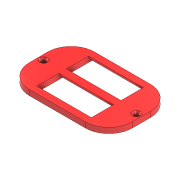
# Autodesk Inventor part: Wago2Din_2Way
Saved by Autodesk Inventor 2021 (Build 250183000, 183)
## iProperties
Created: 2021-07-31
Part Number: Wago2Din_2Way
Material: Generisch
Document SubType Name: Modeling
Designer: Rama
Density: 1 g/cm^3
Appearance: Hellrot
Author: Rama
Autodesk Inventor part; units mm, degrees
ref_plane "YZ Plane" through (0, 0, 0) normal (1, 0, 0) x (0, 1, 0)
ref_plane "XZ Plane" through (0, 0, 0) normal (0, 1, 0) x (-1, 0, 0)
ref_plane "XY Plane" through (0, 0, 0) normal (0, 0, 1) x (1, 0, 0)
sketch "Skizze1" plane through (0, 0, 0) normal (0, 1, 0) x (-1, 0, 0)
  line L0 (15.1, 14.35) -> (-15.1, 14.35)
  line L1 (-15.1, 14.35) -> (-15.1, 2.05)
  line L2 (-15.1, 2.05) -> (15.1, 2.05)
  line L3 (15.1, 2.05) -> (15.1, 14.35)
  line L4 (15.1, 14.35) -> (-15.1, 2.05) construction
  line L5 (-15.1, 14.35) -> (15.1, 2.05) construction
  line L6 (15.1, -2.05) -> (-15.1, -2.05)
  line L7 (-15.1, -2.05) -> (-15.1, -14.35)
  line L8 (-15.1, -14.35) -> (15.1, -14.35)
  line L9 (15.1, -14.35) -> (15.1, -2.05)
  line L10 (15.1, -2.05) -> (-15.1, -14.35) construction
  line L11 (-15.1, -2.05) -> (15.1, -14.35) construction
  line L12 (28.45, 18) -> (-28.45, 18)
  line L13 (-28.45, 18) -> (-28.45, -18)
  line L14 (-28.45, -18) -> (28.45, -18)
  line L15 (28.45, -18) -> (28.45, 18)
  line L16 (28.45, 18) -> (-28.45, -18) construction
  line L17 (-28.45, 18) -> (28.45, -18) construction
  point P0 (0, 0)
  point P1 (0, 8.2)
  point P2 (0, -8.2)
  dimension "d0" = 30.2
  dimension "d1" = 12.3
  dimension "d2" = 30.2
  dimension "d3" = 12.3
  dimension "d5" = 4.1
  dimension "d6" = 2.05
  dimension "d7" = 56.9
  dimension "d8" = 36
  constraints: 36 end point, 6 midpoint, 6 parallel, 3 horizontal, 3 perpendicular
  measures "d0" distance of L2.end L1.end
  measures "d1" distance of L1.end L0.end
  measures "d2" distance of L8.end L7.end
  measures "d3" distance of L7.end L6.end
  measures "d5" distance between parallel lines of L6 L2
  measures "d6" distance from line of point (0, 0) L6
  measures "d7" distance of L14.end L13.end
  measures "d8" distance of L13.end L12.end
extrude "Extrusion1" add sketch "Skizze1" along normal blind 3
chamfer "Fase1" distance 2 angle 45 4 edges at (0, 0, 2.05) (0, 0, -14.35) (0, 0, -2.05) (0, 0, 14.35)
sketch "Skizze2" plane through (0, 3, 0) normal (0, 1, 0) x (1, 0, 0)
  line L0 (28.45, 18) -> (-28.45, 18) projected
  line L1 (-25.65, -18) -> (25.65, -18)
  line L2 (25.65, -18) -> (25.65, 18)
  line L3 (25.65, 18) -> (-25.65, 18)
  line L4 (-25.65, 18) -> (-25.65, -18)
  line L5 (-25.65, -18) -> (25.65, 18) construction
  line L6 (25.65, -18) -> (-25.65, 18) construction
  line L7 (-25.65, 0) -> (25.65, 0)
  point P0 (0, 0)
  dimension "d14" = 51.3
  constraints: 14 end point, 4 midpoint, 2 parallel, 1 horizontal, 1 perpendicular, 1 point on line
  measures "d14" distance of L3.end L2.end
hole "Bohrung1" at (-25.65, 3, 0) at (25.65, 3, 0) direction (0, -1, 0) diameter 2.4 end through all countersink diameter 4.4 countersink angle 90 clearance for "Flachkopfmaschinenschraube" size "M2" standard "ANSI Metrisches M Profil"
fillet "Rundung1" radius 13 4 edges at (28.45, 1.5, -18) (28.45, 1.5, 18) (-28.45, 1.5, -18) (-28.45, 1.5, 18)
